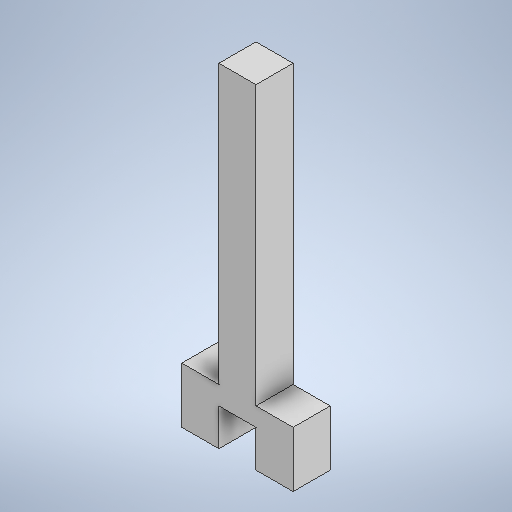
# Autodesk Inventor part: Sorting Holder x2
Saved by Autodesk Inventor 2025.3 (Build 293356000, 356)
## iProperties
Created: 2026-04-19
Part Number: Sorting Holder x2
Material: Generic
Document SubType Name: Modeling
Designer: kamal
Density: 1 g/cm^3
Appearance: Default
Author: kamal
Autodesk Inventor part; units mm, degrees
ref_plane "YZ Plane" through (0, 0, 0) normal (1, 0, 0) x (0, 1, 0)
ref_plane "XZ Plane" through (0, 0, 0) normal (0, 1, 0) x (-1, 0, 0)
ref_plane "XY Plane" through (0, 0, 0) normal (0, 0, 1) x (1, 0, 0)
sketch "Sketch1" plane through (0, 0, 0) normal (0, 0, 1) x (1, 0, 0)
  line L0 (0, 0) -> (0, 90) construction
  line L1 (0, 0) -> (0, 10) construction
  line L2 (0, 10) -> (-5, 10)
  line L3 (-5, 10) -> (-5, 0)
  line L4 (-5, 0) -> (-15, 0)
  line L5 (-15, 0) -> (-15, 10)
  line L6 (-15, 10) -> (-15, 15)
  line L7 (-15, 15) -> (-5, 15)
  line L8 (-5, 15) -> (-5, 90)
  line L9 (-5, 90) -> (0, 90)
  line L10 (0, 10) -> (5, 10)
  line L11 (5, 10) -> (5, 0)
  line L12 (5, 0) -> (15, 0)
  line L13 (15, 0) -> (15, 10)
  line L14 (15, 10) -> (15, 15)
  line L15 (15, 15) -> (5, 15)
  line L16 (5, 15) -> (5, 90)
  line L17 (5, 90) -> (0, 90)
  dimension "d0" = 90
  dimension "d1" = 10
  dimension "d2" = 5
  dimension "d3" = 10
  dimension "d4" = 10
  dimension "d5" = 5
  dimension "d6" = 75
  dimension "d7" = 10
  constraints: 36 end point, 7 symmetric about line, 5 perpendicular, 3 point on line, 3 vertical
  measures "d0" distance of L0.start L0.end
  measures "d1" distance of L0.start L1.end
  measures "d2" distance of L1.end L2.end
  measures "d3" distance of L3.end L4.end
  measures "d4" distance between parallel lines of L4 L2
  measures "d5" distance of L5.end L6.end
  measures "d6" distance of L7.end L8.end
  measures "d7" diameter of L8 L0
extrude "Extrusion1" add sketch "Sketch1" along normal blind 10
body "Solid1"
